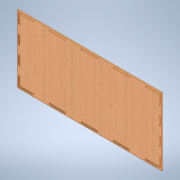
# Autodesk Inventor part: Cara frontal 2
Saved by Autodesk Inventor 2020.3 (Build 243373000, 373)
## iProperties
Created: 2020-04-28
Part Number: Cara frontal 2
Material: Madera (cerezo)
Document SubType Name: Modeling
Designer: miosh
Density: 0.63 g/cm^3
Appearance: Cerezo - Natural brillo bajo
Author: miosh
Autodesk Inventor part; units mm, degrees
ref_plane "YZ Plane" through (0, 0, 0) normal (1, 0, 0) x (0, 1, 0)
ref_plane "XZ Plane" through (0, 0, 0) normal (0, 1, 0) x (-1, 0, 0)
ref_plane "XY Plane" through (0, 0, 0) normal (0, 0, 1) x (1, 0, 0)
sketch "Boceto1" plane through (0, 0, 0) normal (0, 0, 1) x (1, 0, 0)
  line L0 (0, 0) -> (0, 210)
  line L1 (0, 210) -> (450, 210)
  line L2 (450, 210) -> (450, 0)
  line L3 (450, 0) -> (0, 0)
  line L4 (5, 5) -> (50, 5)
  line L5 (50, 5) -> (50, 8)
  line L6 (5, 5) -> (5, 35.71)
  line L7 (5, 35.71) -> (8, 35.71)
  line L8 (50, 8) -> (8, 8)
  line L9 (8, 8) -> (8, 35.71)
  line L10 (5, 63.43) -> (5, 91.14)
  line L11 (5, 118.86) -> (5, 146.57)
  line L12 (5, 174.29) -> (5, 205)
  line L13 (5, 63.43) -> (8, 63.43)
  line L14 (8, 63.43) -> (8, 91.14)
  line L15 (8, 91.14) -> (5, 91.14)
  line L16 (5, 118.86) -> (8, 118.86)
  line L17 (8, 118.86) -> (8, 146.57)
  line L18 (8, 146.57) -> (5, 146.57)
  line L19 (5, 205) -> (50, 205)
  line L20 (50, 205) -> (50, 202)
  line L21 (50, 202) -> (8, 202)
  line L22 (8, 202) -> (8, 174.29)
  line L23 (8, 174.29) -> (5, 174.29)
  line L24 (100, 205) -> (150, 205)
  line L25 (200, 205) -> (250, 205)
  line L26 (300, 205) -> (350, 205)
  line L27 (400, 205) -> (445, 205)
  line L28 (100, 205) -> (100, 202)
  line L29 (100, 202) -> (150, 202)
  line L30 (150, 202) -> (150, 205)
  line L31 (200, 205) -> (200, 202)
  line L32 (200, 202) -> (250, 202)
  line L33 (250, 202) -> (250, 205)
  line L34 (300, 205) -> (300, 202)
  line L35 (300, 202) -> (350, 202)
  line L36 (350, 202) -> (350, 205)
  line L37 (445, 205) -> (445, 174.29)
  line L38 (400, 205) -> (400, 202)
  line L39 (400, 202) -> (442, 202)
  line L40 (442, 202) -> (442, 174.29)
  line L41 (442, 174.29) -> (445, 174.29)
  line L42 (100, 5) -> (150, 5)
  line L43 (200, 5) -> (250, 5)
  line L44 (300, 5) -> (350, 5)
  line L45 (400, 5) -> (445, 5)
  line L46 (100, 5) -> (100, 8)
  line L47 (100, 8) -> (150, 8)
  line L48 (150, 8) -> (150, 5)
  line L49 (200, 5) -> (200, 8)
  line L50 (200, 8) -> (250, 8)
  line L51 (250, 8) -> (250, 5)
  line L52 (300, 5) -> (300, 8)
  line L53 (300, 8) -> (350, 8)
  line L54 (350, 8) -> (350, 5)
  line L55 (445, 5) -> (445, 35.71)
  line L56 (445, 35.71) -> (442, 35.71)
  line L57 (400, 5) -> (400, 8)
  line L58 (400, 8) -> (442, 8)
  line L59 (442, 8) -> (442, 35.71)
  line L60 (445, 63.43) -> (445, 91.14)
  line L61 (445, 118.86) -> (445, 146.57)
  line L62 (445, 63.43) -> (442, 63.43)
  line L63 (442, 63.43) -> (442, 91.14)
  line L64 (442, 91.14) -> (445, 91.14)
  line L65 (445, 118.86) -> (442, 118.86)
  line L66 (442, 118.86) -> (442, 146.57)
  line L67 (442, 146.57) -> (445, 146.57)
  dimension "d0" = 210
  dimension "d1" = 450
  dimension "d2" = 210
  dimension "d3" = 45
  dimension "d4" = 3
  dimension "d5" = 30.71
  dimension "d7" = 42
  dimension "d8" = 3
  dimension "d9" = 27.72
  dimension "d10" = 27.71
  dimension "d11" = 27.72
  dimension "d12" = 27.71
  dimension "d13" = 27.72
  dimension "d14" = 30.71
  dimension "d15" = 3
  dimension "d16" = 27.71
  dimension "d17" = 3
  dimension "d18" = 27.71
  dimension "d19" = 45
  dimension "d20" = 3
  dimension "d21" = 42
  dimension "d22" = 50
  dimension "d23" = 50
  dimension "d24" = 50
  dimension "d25" = 50
  dimension "d26" = 50
  dimension "d27" = 50
  dimension "d28" = 50
  dimension "d29" = 45
  dimension "d31" = 3
  dimension "d32" = 50
  dimension "d33" = 3
  dimension "d34" = 50
  dimension "d35" = 3
  dimension "d36" = 50
  dimension "d37" = 30.71
  dimension "d38" = 3
  dimension "d39" = 42
  dimension "d40" = 50
  dimension "d41" = 50
  dimension "d42" = 50
  dimension "d43" = 50
  dimension "d44" = 50
  dimension "d45" = 50
  dimension "d46" = 50
  dimension "d47" = 45
  dimension "d51" = 3
  dimension "d52" = 50
  dimension "d53" = 3
  dimension "d54" = 50
  dimension "d55" = 3
  dimension "d56" = 50
  dimension "d57" = 30.71
  dimension "d58" = 3
  dimension "d59" = 3
  dimension "d60" = 27.72
  dimension "d61" = 27.71
  dimension "d62" = 27.72
  dimension "d63" = 27.71
  dimension "d64" = 3
  dimension "d65" = 3
  dimension "d69" = 5
  dimension "d71" = 5
  dimension "d72" = 5
  constraints: 136 end point, 23 perpendicular, 19 point on line, 7 parallel, 7 vertical, 3 horizontal
  measures "d0" distance of L0.start L0.end
  measures "d1" distance of L0.end L1.end
  measures "d2" distance of L1.end L2.end
  measures "d3" distance of L4.start L4.end
  measures "d4" distance of L4.end L5.end
  measures "d5" distance of L4.start L6.end
  measures "d7" distance of L5.end L8.end
  measures "d8" distance between parallel lines of L9 L6
  measures "d9" distance of L6.end L10.start
  measures "d10" distance of L10.start L10.end
  measures "d11" distance of L10.end L11.start
  measures "d12" distance of L11.start L11.end
  measures "d13" distance of L11.end L12.start
  measures "d14" distance of L12.start L12.end
  measures "d15" distance of L10.start L13.end
  measures "d16" distance of L13.end L14.end
  measures "d17" distance of L11.start L16.end
  measures "d18" distance of L16.end L17.end
  measures "d19" distance of L12.end L19.end
  measures "d20" distance of L19.end L20.end
  measures "d21" distance of L20.end L21.end
  measures "d22" distance of L19.end L24.start
  measures "d23" distance of L24.start L24.end
  measures "d24" distance of L24.end L25.start
  measures "d25" distance of L25.start L25.end
  measures "d26" distance of L25.end L26.start
  measures "d27" distance of L26.start L26.end
  measures "d28" distance of L26.end L27.start
  measures "d29" distance of L27.start L27.end
  measures "d31" distance of L24.start L28.end
  measures "d32" distance of L28.end L29.end
  measures "d33" distance of L25.start L31.end
  measures "d34" distance of L31.end L32.end
  measures "d35" distance of L26.start L34.end
  measures "d36" distance of L34.end L35.end
  measures "d37" distance of L27.end L37.end
  measures "d38" distance of L27.start L38.end
  measures "d39" distance of L38.end L39.end
  measures "d40" distance of L4.end L42.start
  measures "d41" distance of L42.start L42.end
  measures "d42" distance of L42.end L43.start
  measures "d43" distance of L43.start L43.end
  measures "d44" distance of L43.end L44.start
  measures "d45" distance of L44.start L44.end
  measures "d46" distance of L44.end L45.start
  measures "d47" distance of L45.start L45.end
  measures "d51" distance of L42.start L46.end
  measures "d52" distance of L46.end L47.end
  measures "d53" distance of L43.start L49.end
  measures "d54" distance of L49.end L50.end
  measures "d55" distance of L44.start L52.end
  measures "d56" distance of L52.end L53.end
  measures "d57" distance of L45.end L55.end
  measures "d58" distance of L55.end L56.end
  measures "d59" distance of L45.start L57.end
  measures "d60" distance of L55.end L60.start
  measures "d61" distance of L60.start L60.end
  measures "d62" distance of L60.end L61.start
  measures "d63" distance of L61.start L61.end
  measures "d64" distance of L60.start L62.end
  measures "d65" distance of L61.start L65.end
  measures "d69" distance between parallel lines of L3 L4
  measures "d71" distance between parallel lines of L1 L19
  measures "d72" distance between parallel lines of L27 L1
extrude "Extrusión1" add sketch "Boceto1" along normal blind 3
